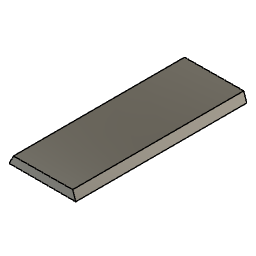
stamp-1 v2 (Autodesk Fusion 360 design; units mm, degrees)
Autodesk Fusion 360 part; units mm, degrees
sketch "Sketch1" plane through (0, 0, 0) normal (0, 1, 0) x (1, 0, 0) in component "plate"
  line L0 (0, 0) -> (35, 0)
  line L1 (35, 0) -> (33.3983, -4.7365)
  line L2 (0, 0) -> (2.2361, -4.4721)
  line L3 (2.2361, -4.4721) -> (33.3983, -4.7365)
  dimension "d1" = 35
  dimension "d2" = 5
  dimension "d4" = 5
  constraint coincident L0.start L2.start
  constraint horizontal L0
  measures "d1" distance of L0.start L0.end
  measures "d2" distance of L0.end L1.end
  measures "d4" distance of L0.start L2.end
extrude "Extrude1" add sketch "Sketch1" along normal blind 90 in component "plate"
component "plate" placed x (1, 0, 0) y (0, 1, 0) z (0, 0, 1) at (0, 0, 0)
